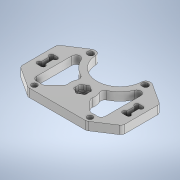
# Autodesk Inventor part: Leg_joint_roll_back_frame
Saved by Autodesk Inventor 2020 (Build 240168000, 168)
## iProperties
Created: 2021-10-17
Part Number: Leg_joint_roll_back_frame
Material: アルミニウム 2014-T4
Document SubType Name: Modeling
Designer: Masato Kubotera
Density: 2.8 g/cm^3
Appearance: 滑らか - 淡い灰色
Description: A2017 T4
Author: Masato Kubotera
Autodesk Inventor part; units mm, degrees
ref_plane "YZ Plane" through (0, 0, 0) normal (1, 0, 0) x (0, 1, 0)
ref_plane "XZ Plane" through (0, 0, 0) normal (0, 1, 0) x (-1, 0, 0)
ref_plane "XY Plane" through (0, 0, 0) normal (0, 0, 1) x (1, 0, 0)
derived "Leg_joint_roll_basis.ipt"
sketch "スケッチ1" plane through (0, 0, 0) normal (0, 0, 1) x (1, 0, 0)
  line L0 (0, 47.48) -> (0, -12.4) construction
  line L1 (-12.5, 47.48) -> (12.5, 47.48) construction
  line L2 (-12.5, 47.48) -> (-12.5, 42.48) construction
  line L3 (-12.5, 42.48) -> (-6.9432, -0.8896) construction
  arc A0 (-6.9432, -0.8896) -> (6.9432, -0.8896) centre (0, 0) ccw construction
  line L4 (-5.51, 45) -> (-3.41, 45) construction
  line L5 (5.51, 45) -> (5.51, 42.48) construction
  line L6 (5.51, 42.48) -> (3.41, 42.48) construction
  line L7 (-5.51, 42.48) -> (-5.51, 45) construction
  line L8 (-5.51, 45) -> (5.51, 42.48) construction
  line L9 (5.51, 45) -> (-5.51, 42.48) construction
  line L10 (-5.5, 44.99) -> (5.5, 44.99) construction
  line L11 (5.5, 44.99) -> (5.5, 42.49) construction
  line L12 (5.5, 42.49) -> (-5.5, 42.49) construction
  line L13 (-5.5, 42.49) -> (-5.5, 44.99) construction
  line L14 (-5.5, 44.99) -> (5.5, 42.49) construction
  line L15 (5.5, 44.99) -> (-5.5, 42.49) construction
  line L16 (-5.51, 43.74) -> (5.51, 43.74) construction
  arc A1 (-3.41, 45) -> (-5.51, 45) centre (-4.46, 45) ccw construction
  arc A2 (-5.51, 42.48) -> (-3.41, 42.48) centre (-4.46, 42.48) ccw construction
  circle A3 centre (-9.5, 45) radius 1.55 construction
  line L17 (12.5, 42.48) -> (6.9432, -0.8896) construction
  line L18 (12.5, 47.48) -> (12.5, 42.48) construction
  circle A4 centre (9.5, 45) radius 1.55 construction
  arc A5 (5.51, 45) -> (3.41, 45) centre (4.46, 45) ccw construction
  arc A6 (3.41, 42.48) -> (5.51, 42.48) centre (4.46, 42.48) ccw construction
  line L19 (-3.41, 45) -> (3.41, 45) construction
  line L20 (-3.41, 42.48) -> (-5.51, 42.48) construction
  line L21 (3.41, 42.48) -> (-3.41, 42.48) construction
  line L22 (3.41, 45) -> (5.51, 45) construction
  circle A7 centre (0, 0) radius 4.05 construction
  line L23 (-13.5, 17) -> (13.5, 17) construction
  line L24 (13.5, 17) -> (13.5, -10) construction
  line L25 (13.5, -10) -> (-13.5, -10) construction
  line L26 (-13.5, -10) -> (-13.5, 17) construction
  line L27 (-13.5, 17) -> (13.5, -10) construction
  line L28 (13.5, 17) -> (-13.5, -10) construction
  arc A8 (-13.5, 18.35) -> (-13.5, 15.65) centre (-13.5, 17) ccw
  circle A9 centre (-13.5, -10) radius 1.35
  line L29 (-24.81, 12.5) -> (-24.81, -5.5)
  circle A10 centre (-13.5, -10) radius 2.4 construction
  line L30 (-24.81, -5.5) -> (-14.2125, -12.4)
  line L31 (-21.75, 7.5) -> (-19.75, 7.5) construction
  line L32 (-19.75, 7.5) -> (-19.75, -0.5) construction
  line L33 (-19.75, -0.5) -> (-21.75, -0.5) construction
  line L34 (-21.75, -0.5) -> (-21.75, 7.5) construction
  line L35 (-21.75, 7.5) -> (-19.75, -0.5) construction
  line L36 (-19.75, 7.5) -> (-21.75, -0.5) construction
  line L37 (-21.76, 7.51) -> (-19.74, 7.51)
  line L38 (-19.74, 7.51) -> (-19.74, 5.41) construction
  line L39 (-19.74, -0.51) -> (-21.76, -0.51)
  line L40 (-21.76, -0.51) -> (-21.76, 1.59) construction
  line L41 (-21.76, 7.51) -> (-19.74, -0.51) construction
  line L42 (-19.74, 7.51) -> (-21.76, -0.51) construction
  arc A11 (-21.76, 7.51) -> (-21.76, 5.41) centre (-21.76, 6.46) ccw
  line L43 (-20.75, 7.51) -> (-20.75, -0.51) construction
  line L44 (-21.76, 3.5) -> (-19.74, 3.5) construction
  arc A12 (-19.74, 5.41) -> (-19.74, 7.51) centre (-19.74, 6.46) ccw
  arc A13 (-21.76, 1.59) -> (-21.76, -0.51) centre (-21.76, 0.54) ccw
  arc A14 (-19.74, -0.51) -> (-19.74, 1.59) centre (-19.74, 0.54) ccw
  line L45 (-24.81, 12.5) -> (-14.2125, 19.4)
  line L46 (-13.5, 18.35) -> (-13, 18.35)
  line L47 (-13.5, 15.65) -> (-13, 15.65)
  arc A15 (-13, 15.65) -> (-13, 18.35) centre (-13, 17) ccw
  line L48 (-21.76, 5.41) -> (-21.76, 7.51) construction
  line L49 (-21.76, 1.59) -> (-21.76, 5.41)
  line L50 (-19.74, 1.59) -> (-19.74, -0.51) construction
  line L51 (-19.74, 5.41) -> (-19.74, 1.59)
  line L52 (19.74, 5.41) -> (19.74, 1.59)
  line L53 (21.76, 1.59) -> (21.76, 5.41)
  arc A16 (21.76, 5.41) -> (21.76, 7.51) centre (21.76, 6.46) ccw
  line L54 (21.76, 7.51) -> (19.74, 7.51)
  arc A17 (19.74, 7.51) -> (19.74, 5.41) centre (19.74, 6.46) ccw
  arc A18 (21.76, -0.51) -> (21.76, 1.59) centre (21.76, 0.54) ccw
  line L55 (19.74, -0.51) -> (21.76, -0.51)
  arc A19 (19.74, 1.59) -> (19.74, -0.51) centre (19.74, 0.54) ccw
  line L56 (24.81, 12.5) -> (24.81, -5.5)
  line L57 (24.81, 12.5) -> (14.2125, 19.4)
  arc A20 (13, 18.35) -> (13, 15.65) centre (13, 17) ccw
  line L58 (13.5, 18.35) -> (13, 18.35)
  arc A21 (13.5, 15.65) -> (13.5, 18.35) centre (13.5, 17) ccw
  line L59 (24.81, -5.5) -> (14.2125, -12.4)
  circle A22 centre (13.5, -10) radius 1.35
  line L60 (13.5, 15.65) -> (13, 15.65)
  line L61 (-14.2125, -12.4) -> (14.2125, -12.4)
  line L62 (-14.2125, 19.4) -> (-11.0486, 19.4)
  circle A23 centre (0, 18) radius 5.05 construction
  circle A24 centre (-13.5, 17) radius 2.4 construction
  arc A25 (-11.0486, 19.4) -> (11.0486, 19.4) centre (0, 18) ccw
  line L63 (11.0486, 19.4) -> (14.2125, 19.4)
  circle A26 centre (0, 26.5) radius 1.35 construction
  circle A27 centre (-8.5, 18) radius 1.35 construction
  circle A28 centre (0, 9.5) radius 1.35 construction
  circle A29 centre (8.5, 18) radius 1.35 construction
  arc A30 (-10.4884, 20.9672) -> (10.4884, 20.9672) centre (0, 18) ccw construction
  arc A31 (5.7734, 37.6333) -> (-5.7734, 37.6333) centre (0, 36) ccw construction
  line L64 (-5.7734, 37.6333) -> (-10.4884, 20.9672) construction
  line L65 (5.7734, 37.6333) -> (10.4884, 20.9672) construction
  circle A32 centre (0, 36) radius 2.25 construction
  circle A33 centre (0, 9.5) radius 2.4 construction
  circle A34 centre (0, 0) radius 2.25
  circle A35 centre (0, 0) radius 1.55
  line L66 (0, -3.187) -> (-0.9093, -2.662) construction
  line L67 (-2.76, -1.5935) -> (-2.76, -0.5435) construction
  line L68 (-2.76, 1.5935) -> (-1.8507, 2.1185) construction
  line L69 (0, 3.187) -> (2.76, 1.5935)
  line L70 (2.76, 1.5935) -> (2.76, 0.5435) construction
  line L71 (2.76, -1.5935) -> (1.8507, -2.1185) construction
  arc A36 (0.9093, 2.662) -> (-0.9093, 2.662) centre (0, 2.137) ccw
  arc A37 (-1.8507, 2.1185) -> (-2.76, 0.5435) centre (-1.8507, 1.0685) ccw
  arc A38 (-2.76, -0.5435) -> (-1.8507, -2.1185) centre (-1.8507, -1.0685) ccw
  arc A39 (-0.9093, -2.662) -> (0.9093, -2.662) centre (0, -2.137) ccw
  arc A40 (1.8507, -2.1185) -> (2.76, -0.5435) centre (1.8507, -1.0685) ccw
  arc A41 (2.76, 0.5435) -> (1.8507, 2.1185) centre (1.8507, 1.0685) ccw
  line L72 (-0.9093, 2.662) -> (0, 3.187) construction
  line L73 (-1.8507, 2.1185) -> (-0.9093, 2.662)
  line L74 (-2.76, 0.5435) -> (-2.76, 1.5935) construction
  line L75 (-2.76, -0.5435) -> (-2.76, 0.5435)
  line L76 (-1.8507, -2.1185) -> (-2.76, -1.5935) construction
  line L77 (-0.9093, -2.662) -> (-1.8507, -2.1185)
  line L78 (0.9093, -2.662) -> (0, -3.187) construction
  line L79 (1.8507, -2.1185) -> (0.9093, -2.662)
  line L80 (2.76, -0.5435) -> (2.76, -1.5935) construction
  line L81 (2.76, 0.5435) -> (2.76, -0.5435)
  circle A42 centre (0, 0) radius 3 construction
  line L82 (-16.75, 14.168) -> (-16.75, -7.168)
  line L83 (-16.75, 14.168) -> (-15.12, 15.2292)
  arc A43 (-15.12, 15.2292) -> (-13.7246, 14.6105) centre (-13.5, 17) ccw
  line L84 (-16.75, -7.168) -> (-15.12, -8.2292)
  arc A44 (-4.0263, 4.4485) -> (-5.6149, -2.1149) centre (0, 0) ccw
  arc A45 (-13.7246, 14.6105) -> (-4.0263, 4.4485) centre (0, 18) ccw
  line L85 (-5.6149, -2.1149) -> (-11.8029, -8.3029)
  arc A46 (-11.8029, -8.3029) -> (-15.12, -8.2292) centre (-13.5, -10) ccw
  line L86 (16.75, 14.168) -> (16.75, -7.168)
  line L87 (16.75, 14.168) -> (15.12, 15.2292)
  arc A47 (13.7246, 14.6105) -> (15.12, 15.2292) centre (13.5, 17) ccw
  line L88 (16.75, -7.168) -> (15.12, -8.2292)
  arc A48 (5.6149, -2.1149) -> (4.0263, 4.4485) centre (0, 0) ccw
  arc A49 (4.0263, 4.4485) -> (13.7246, 14.6105) centre (0, 18) ccw
  line L89 (5.6149, -2.1149) -> (11.8029, -8.3029)
  arc A50 (15.12, -8.2292) -> (11.8029, -8.3029) centre (13.5, -10) ccw
  point P0 (0, 43.74)
  point P1 (0, 3.5)
  point P2 (-20.75, 3.5)
  point P3 (-24.81, 3.5)
  point P4 (-13.5, 3.5)
  point P5 (1.8507, 2.1185)
  dimension "d1" = 3
  dimension "d2" = 3
  dimension "d4" = 3
  dimension "d5" = 6
  measures "d1" distance between parallel lines of L45 L83
  measures "d2" distance between parallel lines of L82 L32
  measures "d4" radial gap between concentric circles of A45 A25
  measures "d5" radius of A44
extrude "押し出し1" add sketch "スケッチ1" along normal blind 4 contours L45 L62 A25 L63 L57 L56 L59 L61 L30 L29
extrude "押し出し2" add sketch "スケッチ1" along normal blind 1.8 contours A36 L69 | L69 A41 L81 A40 L79 A39 L77 A38 L75 A37 L73 A36 | A41 L69
fillet "フィレット1" radius 2 10 edges at (14.2125, 19.4, 2) (11.0486, 19.4, 2) (24.81, 12.5, 2) (24.81, -5.5, 2) (14.2125, -12.4, 2) (-14.2125, -12.4, 2) (-24.81, -5.5, 2) (-24.81, 12.5, 2) (-14.2125, 19.4, 2) (-11.0486, 19.4, 2)
fillet "フィレット2" radius 2 16 edges at (-13.7246, 14.6105, 2) (-15.12, 15.2292, 2) (-16.75, 14.168, 2) (-4.0263, 4.4485, 2) (-5.6149, -2.1149, 2) (-11.8029, -8.3029, 2) (-15.12, -8.2292, 2) (-16.75, -7.168, 2) (5.6149, -2.1149, 2) (4.0263, 4.4485, 2) (13.7246, 14.6105, 2) (15.12, 15.2292, 2) (16.75, 14.168, 2) (16.75, -7.168, 2) (15.12, -8.2292, 2) (11.8029, -8.3029, 2)
extrude "押し出し3" add sketch "スケッチ1" along normal blind 1 contours A34
equation "\"d2\" = d1"
equation "\"d4\" = d1"
equation "\"d3\" = d1"
